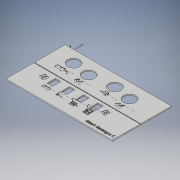
# Autodesk Inventor part: Caixa control - tapa
Saved by Autodesk Inventor 2019 (Build 230136000, 136)
## iProperties
Created: 2018-08-29
Part Number: Caixa control - tapa
Material: Genérico
Document SubType Name: Modeling
Designer: Albert Garangou Culebras
Density: 1 g/cm^3
Appearance: Valor por defecto
Author: Albert Garangou Culebras
Autodesk Inventor part; units mm, degrees
(part 1 of 2)
ref_plane "YZ Plane" through (0, 0, 0) normal (1, 0, 0) x (0, 1, 0)
ref_plane "XZ Plane" through (0, 0, 0) normal (0, 1, 0) x (-1, 0, 0)
ref_plane "XY Plane" through (0, 0, 0) normal (0, 0, 1) x (1, 0, 0)
sketch "Boceto1" plane through (0, 0, 0) normal (0, 1, 0) x (-1, 0, 0)
  line L0 (0, 0) -> (-180, 0)
  line L1 (-180, 0) -> (-180, -100)
  line L2 (-180, -100) -> (0, -100)
  line L3 (0, -100) -> (0, 0)
  dimension "d0" = 180
  dimension "d1" = 100
  constraints: 8 end point, 2 parallel, 1 horizontal, 1 perpendicular
  measures "d0" distance of L2.end L1.end
  measures "d1" distance of L1.end L0.end
extrude "base" add sketch "Boceto1" along normal blind 2
sketch "Boceto2" plane through (0, 2, 0) normal (0, 1, 0) x (1, 0, 0)
  line L0 (0, 100) -> (0, 0) projected
  line L1 (0, 0) -> (180, 0) projected
  line L2 (0, 100) -> (180, 100)
  line L3 (180, 100) -> (180, 0)
  line L4 (180, 0) -> (0, 0)
  line L5 (0, 0) -> (0, 100)
  line L6 (180, 50) -> (180, 0)
  line L7 (180, 0) -> (84.2308, 0)
  line L8 (180, 100) -> (0, 100) projected
  circle A0 centre (34.2888, 79.9235) radius 10.25
  circle A1 centre (104.2888, 79.9235) radius 10.25
  line L9 (50.4618, 35) -> (50.4618, 42)
  line L10 (50.4618, 42) -> (41.4618, 42)
  line L11 (41.4618, 42) -> (41.4618, 28)
  line L12 (41.4618, 28) -> (50.4618, 28)
  line L13 (50.4618, 28) -> (50.4618, 36)
  line L14 (65.4618, 35) -> (65.4618, 42)
  line L15 (65.4618, 42) -> (74.4618, 42)
  line L16 (74.4618, 42) -> (74.4618, 28)
  line L17 (74.4618, 28) -> (65.4618, 28)
  line L18 (65.4618, 28) -> (65.4618, 35)
  line L19 (89.4618, 35) -> (89.4618, 42)
  line L20 (89.4618, 42) -> (98.4618, 42)
  line L21 (98.4618, 42) -> (98.4618, 28)
  line L22 (98.4618, 28) -> (89.4618, 28)
  line L23 (89.4618, 28) -> (89.4618, 35)
  line L24 (113.4618, 42) -> (122.4618, 42)
  line L25 (122.4618, 42) -> (122.4618, 28)
  line L26 (122.4618, 28) -> (113.4618, 28)
  line L27 (113.4618, 28) -> (113.4618, 42)
  circle A2 centre (64.2888, 75.4263) radius 10.25
  circle A3 centre (134.2888, 74.9235) radius 10.25
  constraints: 50 end point, 11 perpendicular, 4 centre point, 4 parallel, 4 vertical, 3 horizontal, 3 point on line
sketch "Boceto3" plane through (0, 2, 0) normal (0, 1, 0) x (1, 0, 0)
  line L0 (35.7041, 64.3419) -> (35.7041, 63.6919)
  line L1 (35.7042, 59.1622) -> (35.7042, 59.8122)
  line L2 (37.6679, 61.7621) -> (37.6747, 62.4121)
  line L3 (37.6747, 62.4121) -> (38.9746, 62.3985)
  line L4 (37.6679, 61.7621) -> (37.6612, 61.1121)
  line L5 (37.6612, 61.1121) -> (38.961, 61.0986)
  line L6 (41.5539, 61.0919) -> (42.8539, 61.0919) construction
  line L7 (42.8539, 61.0919) -> (42.8539, 58.4716) construction
  spline S0 degree 2 poles (41.5539, 61.0919) (42.8539, 61.0919) (42.8539, 58.4716) knots 1 1 1 2 2 2
  line L8 (41.554, 62.3716) -> (44.1539, 62.3716) construction
  line L9 (44.1539, 62.3716) -> (44.1539, 58.4716) construction
  spline S1 degree 2 poles (41.554, 62.3716) (44.1539, 62.3716) (44.1539, 58.4716) knots 1 1 1 2 2 2
  line L10 (38.954, 61.0919) -> (41.554, 61.0919)
  line L11 (38.9541, 62.3919) -> (41.554, 62.3716)
  line L12 (37.6542, 60.4419) -> (35.7042, 60.4622)
  line L13 (37.6813, 63.0419) -> (35.7041, 63.0419)
  line L14 (37.6813, 63.0419) -> (37.6747, 62.4121)
  line L15 (37.6612, 61.1121) -> (37.6542, 60.4419)
  line L16 (42.8539, 57.8216) -> (44.1539, 57.8216)
  line L17 (44.1539, 57.8216) -> (44.1539, 58.4716)
  line L18 (44.1539, 57.8216) -> (43.8939, 57.8216)
  line L19 (42.8539, 58.4716) -> (42.8539, 57.8216)
  line L20 (58.9613, 57.27) -> (63.5735, 61.1094)
  line L21 (64.2117, 60.8104) -> (64.2117, 53.2631)
  line L22 (58.9754, 56.8292) -> (63.5531, 52.9999)
  arc A0 (63.5531, 52.9999) -> (64.2117, 53.2631) centre (63.7962, 53.3472) ccw
  arc A1 (64.2117, 60.8104) -> (63.5735, 61.1094) centre (63.7975, 60.7568) ccw
  arc A2 (58.9613, 57.27) -> (58.9754, 56.8292) centre (59.2258, 57.0578) ccw
  line L23 (64.4328, 57.3171) -> (69.0449, 61.1564)
  line L24 (69.6831, 60.8575) -> (69.6831, 53.3101)
  line L25 (64.4468, 56.8762) -> (69.0245, 53.0469)
  arc A3 (69.0245, 53.0469) -> (69.6831, 53.3101) centre (69.2676, 53.3943) ccw
  arc A4 (69.6831, 60.8575) -> (69.0449, 61.1564) centre (69.2689, 60.8039) ccw
  arc A5 (64.4328, 57.3171) -> (64.4468, 56.8762) centre (64.6972, 57.1049) ccw
  line L26 (58.9613, 57.27) -> (63.5735, 61.1094)
  line L27 (64.2117, 60.8104) -> (64.2117, 53.2631)
  line L28 (58.9754, 56.8292) -> (63.5531, 52.9999)
  arc A6 (58.9613, 57.27) -> (58.9754, 56.8292) centre (59.2258, 57.0578) ccw
  line L29 (69.6831, 60.8575) -> (69.6831, 53.3101)
  line L30 (64.4328, 57.3171) -> (69.0449, 61.1564)
  line L31 (64.4468, 56.8762) -> (69.0245, 53.0469)
  arc A7 (64.4328, 57.3171) -> (64.4468, 56.8762) centre (64.6972, 57.1049) ccw
  line L32 (128.7561, 56.7254) -> (133.3696, 60.5658)
  line L33 (134.0065, 60.2673) -> (134.0065, 52.7184)
  line L34 (128.7702, 56.2845) -> (133.3479, 52.4552)
  arc A8 (133.3479, 52.4552) -> (134.0065, 52.7184) centre (133.591, 52.8025) ccw
  arc A9 (128.7561, 56.7254) -> (128.7702, 56.2845) centre (129.0205, 56.5132) ccw
  line L35 (139.4779, 60.3128) -> (139.4779, 52.7655)
  arc A10 (138.8193, 52.5023) -> (139.4779, 52.7655) centre (139.0624, 52.8496) ccw
  line L36 (134.2275, 56.7724) -> (138.8397, 60.6118)
  line L37 (134.2416, 56.3316) -> (138.8193, 52.5023)
  arc A11 (134.2275, 56.7724) -> (134.2416, 56.3316) centre (134.4919, 56.5602) ccw
  arc A12 (134.0065, 60.2673) -> (133.3696, 60.5658) centre (133.618, 60.2673) ccw
  arc A13 (139.4779, 60.3128) -> (138.8397, 60.6118) centre (139.0799, 60.294) ccw
  arc A14 (101.959, 62.5573) -> (101.9701, 63.0852) centre (105.955, 62.7371) ccw
  spline S2 degree 3 poles (101.9701, 63.0852) (100.3792, 62.5267) (98.8482, 62.1984) (96.8436, 62.2447) knots 0 0 0 0 1 1 1 1
  circle A15 centre (105.955, 62.7371) radius 1
  arc A16 (108.9509, 62.892) -> (106.5532, 65.6768) centre (105.955, 62.7371) ccw
  line L38 (109.0736, 62.5385) -> (108.7201, 62.892)
  line L39 (109.0736, 62.5385) -> (109.4272, 62.892)
  arc A17 (109.2013, 62.892) -> (106.5532, 65.9315) centre (105.955, 62.7371) ccw
  line L40 (109.4272, 62.892) -> (109.2013, 62.892)
  line L41 (108.9509, 62.892) -> (108.7201, 62.892)
  line L42 (102.8865, 63.4069) -> (101.0538, 62.7635) construction
  arc A18 (101.2329, 62.8412) -> (102.6981, 63.3556) centre (94.8232, 83.4427) ccw construction
  line L43 (96.8436, 62.2447) -> (97.002, 61.7465)
  line L44 (106.5532, 65.9315) -> (106.5532, 65.6768)
  line L45 (35.7041, 64.3419) -> (35.7041, 64.4719)
  line L46 (35.7041, 64.3419) -> (35.7041, 65.6419)
  line L47 (35.7041, 65.6419) -> (33.7541, 65.6419)
  line L48 (33.7541, 65.6419) -> (33.7541, 64.3419)
  line L49 (33.7541, 64.3419) -> (22.7041, 64.3419)
  line L50 (22.7041, 59.1419) -> (22.7041, 64.3419)
  line L51 (33.7541, 59.1419) -> (33.7541, 57.8419)
  line L52 (33.7541, 57.8419) -> (35.704, 57.8419)
  line L53 (35.7042, 57.8419) -> (35.7042, 59.1622)
  line L54 (33.7541, 59.1419) -> (22.7041, 59.1419)
  line L55 (51.2122, 23.1412) -> (51.2122, 22.6162)
  line L56 (51.2122, 18.9576) -> (51.2122, 19.4826)
  line L57 (52.7873, 20.0076) -> (51.2122, 20.0076)
  line L58 (52.7872, 22.0912) -> (51.2122, 22.0912)
  line L59 (52.7872, 22.0912) -> (52.7872, 21.599)
  line L60 (52.7873, 20.549) -> (52.7873, 20.0076)
  line L61 (51.2122, 23.1412) -> (51.2122, 23.2462)
  line L62 (51.2122, 23.1412) -> (51.2122, 24.1912)
  line L63 (51.2122, 24.1912) -> (49.6372, 24.1912)
  line L64 (49.6372, 24.1912) -> (49.6372, 23.1412)
  line L65 (49.6372, 23.1412) -> (40.7122, 23.1412)
  line L66 (40.7122, 18.9412) -> (40.7122, 23.1412)
  line L67 (49.6372, 18.9412) -> (49.6372, 17.8912)
  line L68 (49.6372, 17.8912) -> (51.2122, 17.8912)
  line L69 (51.2122, 17.8912) -> (51.2122, 18.9576)
  line L70 (49.6372, 18.9412) -> (40.7122, 18.9412)
  line L71 (51.2122, 20.0076) -> (51.2122, 19.4826)
  line L72 (51.2122, 22.0912) -> (51.2122, 22.6162)
  line L73 (35.7042, 60.4622) -> (35.7042, 59.8122)
  line L74 (35.7041, 63.6919) -> (35.7041, 63.0419)
  line L75 (52.7872, 21.374) -> (52.4873, 21.374)
  line L76 (52.4873, 21.374) -> (52.4873, 20.774)
  line L77 (52.4873, 20.774) -> (52.7873, 20.774)
  line L78 (52.7873, 20.774) -> (52.7873, 20.549)
  line L79 (52.7872, 21.599) -> (52.7872, 21.374)
  line L80 (89.627, 23.9855) -> (97.277, 23.9855)
  line L81 (97.277, 16.3355) -> (89.627, 16.3355)
  line L82 (89.627, 16.3355) -> (89.627, 23.9855)
  line L83 (67.3452, 22.5763) -> (66.2952, 22.5763)
  line L84 (66.2952, 22.5763) -> (66.2952, 21.8763)
  line L85 (67.3452, 21.8763) -> (67.3452, 22.5763)
  line L86 (67.3452, 21.8763) -> (67.3452, 21.9463)
  line L87 (67.3452, 21.8763) -> (67.3452, 21.5263)
  line L88 (68.3953, 21.1763) -> (67.3452, 21.1763)
  line L89 (68.3953, 19.7747) -> (67.3452, 19.7763)
  line L90 (67.3452, 19.0763) -> (67.3452, 19.4263)
  line L91 (67.3452, 18.3653) -> (67.3452, 19.0763)
  line L92 (66.2952, 19.0749) -> (66.2952, 18.3749)
  line L93 (66.2952, 18.3749) -> (67.3452, 18.3749)
  line L94 (68.3953, 20.1357) -> (68.3953, 19.7747)
  line L95 (67.3452, 19.7763) -> (67.3452, 19.4263)
  line L96 (67.3452, 21.1763) -> (67.3452, 21.5263)
  line L97 (68.3953, 20.2857) -> (68.3953, 20.1357)
  line L98 (68.3953, 21.1763) -> (68.3953, 20.7878)
  line L99 (65.2366, 21.8749) -> (65.2366, 19.0749)
  line L100 (65.2366, 21.8763) -> (66.2952, 21.8763)
  line L101 (65.2366, 19.0749) -> (66.2952, 19.0749)
  line L102 (97.277, 23.9855) -> (97.277, 20.798)
  line L103 (97.277, 19.523) -> (97.277, 16.3355)
  line L104 (100.5679, 20.798) -> (100.5679, 19.523)
  line L105 (100.5679, 19.523) -> (97.277, 19.523)
  line L106 (97.277, 20.798) -> (100.5679, 20.798)
  line L107 (122.2298, 31.1299) -> (122.2298, 16.1299)
  line L108 (122.2298, 16.1299) -> (113.2298, 16.1299)
  line L109 (113.2298, 26.1299) -> (113.2298, 21.1299)
  line L110 (113.2298, 26.1299) -> (113.2298, 25.6299)
  line L111 (113.2298, 21.1299) -> (113.2298, 21.6299)
  line L112 (113.2298, 21.6299) -> (113.2298, 20.6299)
  line L113 (113.2298, 16.1299) -> (114.2298, 16.1299)
  line L114 (122.2298, 16.1299) -> (121.2298, 16.1299)
  line L115 (113.2298, 16.1299) -> (113.2298, 17.1299)
  line L116 (114.2298, 25.6299) -> (121.2298, 25.6299)
  line L117 (121.2298, 25.6299) -> (121.2298, 21.6299)
  line L118 (121.2298, 21.6299) -> (114.2298, 21.6299)
  line L119 (114.2298, 21.6299) -> (114.2298, 25.6299)
  line L120 (114.2298, 20.6299) -> (121.2298, 20.6299)
  line L121 (121.2298, 20.6299) -> (121.2298, 17.1299)
  line L122 (121.2298, 17.1299) -> (114.2298, 17.1299)
  line L123 (114.2298, 17.1299) -> (114.2298, 20.6299)
  line L124 (114.2298, 17.1299) -> (116.5298, 17.1299)
  line L125 (116.5298, 17.1299) -> (118.8298, 17.1299)
  line L126 (117.6798, 17.1299) -> (118.7948, 17.1299)
  line L127 (118.7948, 17.1299) -> (119.9098, 17.1299)
  line L128 (119.9098, 17.1299) -> (121.0248, 17.1299)
  circle A19 centre (120.4673, 19.4799) radius 0.45
  circle A20 centre (118.8673, 19.4799) radius 0.45
  circle A21 centre (117.2673, 19.4799) radius 0.45
  circle A22 centre (118.8673, 24.2799) radius 0.45
  circle A23 centre (120.4673, 24.2799) radius 0.45
  circle A24 centre (117.2673, 24.2799) radius 0.45
  circle A25 centre (118.8673, 29.0799) radius 0.45
  circle A26 centre (120.4673, 29.0799) radius 0.45
  circle A27 centre (117.2673, 29.0799) radius 0.45
  line L129 (114.2298, 17.1299) -> (114.2298, 18.1299)
  line L130 (114.2298, 17.1299) -> (114.9798, 17.1299)
  line L131 (114.9823, 17.6299) -> (117.0198, 17.6299)
  line L132 (117.0198, 17.6299) -> (117.0198, 18.1299)
  line L133 (117.0198, 18.1299) -> (114.9823, 18.1299)
  line L134 (114.9823, 18.1299) -> (114.9823, 17.6299)
  line L135 (114.9823, 22.6299) -> (114.9823, 22.1299)
  line L136 (114.9823, 22.1299) -> (117.0198, 22.1299)
  line L137 (117.0198, 22.6299) -> (114.9823, 22.6299)
  line L138 (117.0198, 22.1299) -> (117.0198, 22.6299)
  line L139 (114.9823, 27.6299) -> (114.9823, 27.1299)
  line L140 (117.0198, 27.6299) -> (114.9823, 27.6299)
  line L141 (117.0198, 27.1299) -> (117.0198, 27.6299)
  line L142 (114.9823, 27.1299) -> (117.0198, 27.1299)
  line L143 (121.2298, 30.6299) -> (121.2298, 26.6299)
  line L144 (40.7122, 23.1412) -> (40.7122, 18.9412)
  line L145 (49.6372, 18.9412) -> (40.7122, 18.9412)
  line L146 (49.6372, 18.9412) -> (49.6372, 17.8912)
  line L147 (49.6372, 17.8912) -> (51.2122, 17.8912)
  line L148 (51.2122, 17.8912) -> (51.2122, 20.0076)
  line L149 (51.2122, 20.0076) -> (52.7873, 20.0076)
  line L150 (52.7873, 20.0076) -> (52.7873, 20.774)
  line L151 (52.7873, 20.774) -> (52.4873, 20.774)
  line L152 (52.4873, 20.774) -> (52.4873, 21.3799)
  line L153 (52.4873, 21.3799) -> (52.7872, 21.3799)
  line L154 (52.7872, 21.3799) -> (52.7872, 22.0908)
  line L155 (52.7872, 22.0908) -> (51.2122, 22.0908)
  line L156 (51.2122, 22.0908) -> (51.2122, 24.1912)
  line L157 (49.6372, 24.1912) -> (51.2122, 24.1912)
  line L158 (49.6372, 24.1912) -> (49.6372, 23.1412)
  line L159 (49.6372, 23.1412) -> (40.7122, 23.1412)
  line L160 (40.7122, 23.1412) -> (40.7122, 18.9412)
  line L161 (22.7041, 64.3419) -> (22.7041, 59.1419)
  line L162 (22.7041, 59.1419) -> (33.7541, 59.1419)
  line L163 (33.7541, 57.8419) -> (33.7541, 59.1419)
  line L164 (33.7541, 57.8419) -> (35.7042, 57.8419)
  line L165 (35.7042, 57.8419) -> (35.7042, 60.4622)
  line L166 (35.7042, 60.4622) -> (37.6542, 60.4419)
  line L167 (37.6542, 60.4419) -> (37.6612, 61.1121)
  line L168 (37.6612, 61.1121) -> (37.6813, 63.0419)
  line L169 (37.6813, 63.0419) -> (35.7041, 63.0419)
  line L170 (35.7041, 63.0419) -> (35.7041, 65.6419)
  line L171 (35.7041, 65.6419) -> (33.7541, 65.6419)
  line L172 (33.7541, 65.6419) -> (33.7541, 64.3419)
  line L173 (33.7541, 64.3419) -> (22.7041, 64.3419)
  line L174 (22.7041, 64.3419) -> (22.7041, 59.1419)
  line L175 (42.8539, 57.8216) -> (44.1539, 57.8216)
  line L176 (44.1539, 58.4716) -> (44.1539, 57.8216)
  line L177 (42.8539, 58.4716) -> (42.8539, 57.8216)
  line L178 (41.554, 61.0919) -> (42.8539, 61.0919) construction
  line L179 (42.8539, 61.0919) -> (42.8539, 58.4716) construction
  spline S3 degree 2 poles (41.554, 61.0919) (42.8539, 61.0919) (42.8539, 58.4716) knots 1 1 1 2 2 2
  line L180 (41.554, 62.3716) -> (44.1539, 62.3716) construction
  line L181 (44.1539, 62.3716) -> (44.1539, 58.4716) construction
  spline S4 degree 2 poles (41.554, 62.3716) (44.1539, 62.3716) (44.1539, 58.4716) knots 1 1 1 2 2 2
  line L182 (65.2366, 21.8763) -> (65.2366, 19.0749)
  line L183 (66.2952, 19.0749) -> (65.2366, 19.0749)
  line L184 (66.2952, 19.0749) -> (66.2952, 18.3749)
  line L185 (66.2952, 18.3749) -> (67.3452, 18.3749)
  line L186 (67.3452, 18.3749) -> (67.3452, 19.7763)
  line L187 (67.3452, 19.7763) -> (68.3953, 19.7747)
  line L188 (68.3953, 20.2857) -> (68.3953, 19.7747)
  line L189 (68.3953, 20.7878) -> (68.3953, 21.1763)
  line L190 (68.3953, 21.1763) -> (67.3452, 21.1763)
  line L191 (67.3452, 21.1763) -> (67.3452, 22.5763)
  line L192 (67.3452, 22.5763) -> (66.2952, 22.5763)
  line L193 (66.2952, 22.5763) -> (66.2952, 21.8763)
  line L194 (66.2952, 21.8763) -> (65.2366, 21.8763)
  line L195 (65.2366, 21.8763) -> (65.2366, 19.0749)
  spline S5 degree 3 poles (68.3953, 20.7878) (70.7304, 20.7878) (70.1192, 19.8403) (75.3334, 20.4894) knots 0 0 0 0 1 1 1 1
  line L196 (75.3828, 20.0925) -> (75.3334, 20.4894)
  line L197 (91.5068, 17.6299) -> (92.143, 17.6299)
  line L198 (92.143, 17.6299) -> (92.143, 22.0105)
  line L199 (92.143, 22.0105) -> (93.452, 19.0299)
  line L200 (93.452, 19.0299) -> (93.8546, 19.0299)
  line L201 (93.8546, 19.0299) -> (95.1799, 22.0105)
  line L202 (95.1799, 22.0105) -> (95.1799, 17.6299)
  line L203 (95.1799, 17.6299) -> (95.8762, 17.6299)
  line L204 (95.8762, 17.6299) -> (95.8762, 22.7264)
  line L205 (94.9375, 22.7264) -> (93.6941, 19.9299)
  line L206 (93.6941, 19.9299) -> (92.4659, 22.7264)
  line L207 (91.5068, 22.7264) -> (92.4659, 22.7264)
  line L208 (91.5068, 22.7264) -> (91.5068, 17.6299)
  line L209 (94.9375, 22.7264) -> (95.8762, 22.7264)
  line L210 (113.2298, 20.6299) -> (113.2298, 17.1299)
  line L211 (114.2298, 26.6299) -> (113.2298, 26.6299)
  line L212 (113.2298, 26.6299) -> (113.2298, 26.1299)
  line L213 (114.2298, 26.6299) -> (122.2298, 26.6299)
  line L214 (37.6612, 61.1121) -> (37.6747, 62.4121)
  line L215 (68.3953, 20.7878) -> (68.3953, 20.3878)
  line L216 (68.3953, 20.3878) -> (68.3953, 19.7747)
  spline S6 degree 5 poles (101.959, 62.5573) (101.0032, 62.2312) (100.028, 61.9616) (99.0225, 61.7956) (98.0118, 61.7336) (97.002, 61.7465) knots 0 0 0 0 0 0 1 1 1 1 1 1
  spline S7 degree 5 poles (68.3953, 20.3878) (68.7147, 20.3874) (69.0333, 20.3731) (69.3537, 20.3357) (70.0075, 20.1748) (70.6566, 19.9957) (71.0075, 19.9367) (72.0927, 19.8215) (73.1869, 19.8682) (73.9195, 19.924) (74.6525, 20.0016) (75.3828, 20.0925) knots 0 0 0 0 0 0 0.226556 0.226556 0.226556 0.477707 0.477707 0.477707 1 1 1 1 1 1
  point P0 (0, 0)
  point P1 (126.2308, 70)
  point P2 (69.8531, 20.6216)
  point P3 (70.8387, 20.3848)
  point P4 (117.6798, 19.4799)
  point P5 (117.6798, 24.2799)
  point P6 (117.6798, 29.0799)
  dimension "d288" = 0.4
  dimension "d259" = 1.6
  dimension "d266" = 4.8
  dimension "d276" = 4.5
  dimension "d283" = 5
  dimension "d289" = 1
  constraints: 418 end point, 42 vertical, 36 collinear, 35 point on circle, 34 perpendicular, 28 centre point, 20 point on line, 12 horizontal, 11 parallel, 5 coincident, 3 midpoint, 1 tangent, 64 other
  measures "d259" distance of A19.centre A20.centre
  measures "d266" distance of A21.centre A24.centre
  measures "d276" distance of L131.start L135.end
  measures "d283" distance of L135.start L139.start
  measures "d289" distance of L116.start L211.start
extrude "Extrusión3" cut sketch "Boceto3" against normal blind 0.5 contours L0 L74 L13 L14 L2 L4 L15 L12 L73 L1 L53 L52 L51 L54 L50 L49 L48 L47 L46 L45 | L20 A1 L21 A0 L22 A2 | L23 A4 L24 A3 L25 A5 | L32 A12 L33 A8 L34 A9 | L35 A10 L37 A11 L36 A13 | S6 L43 S2 A14 | L55 L72 L58 L59 L79 L153 L152 L76 L77 L78 L60 L57 L71 L56 L69 L68 L67 L70 L66 L65 L64 L63 L62 L61 | L80 L102 L106 L104 L105 L103 L81 L82 | L85 L87 L96 L88 L98 L215 L216 L97 L94 L89 L95 L90 L91 L93 L92 L101 L99 L100 L84 L83 | S5 L196 S7 L215 | L107 L108 L115 L210 L112 L109 L212 L211 L213 | A19 | A20 | A21 | A22 | A23 | A24 | L134 L133 L132 L131 | L137 L138 L136 L135
sketch "Boceto5" plane through (0, 2, 0) normal (0, 1, 0) x (1, 0, 0)
  line L0 (37.6813, 63.0419) -> (37.6542, 60.4419) projected
  line L1 (37.6747, 62.4093) -> (37.6612, 61.1175)
  line L2 (41.6533, 62.4093) -> (37.6747, 62.4093)
  line L3 (41.6533, 62.4093) -> (44.1386, 62.4093) construction
  line L4 (44.1386, 62.4093) -> (44.1386, 58.5428) construction
  spline S0 degree 2 poles (41.6533, 62.4093) (44.1386, 62.4093) (44.1386, 58.5428) knots 1 1 1 2 2 2
  line L5 (41.6533, 61.1175) -> (42.896, 61.1175) construction
  line L6 (42.896, 61.1175) -> (42.896, 58.5428) construction
  spline S1 degree 2 poles (41.6533, 61.1175) (42.896, 61.1175) (42.896, 58.5428) knots 1 1 1 2 2 2
  line L7 (42.896, 58.5428) -> (44.1386, 58.5428)
  line L8 (37.6612, 61.1175) -> (41.6533, 61.1175)
  point P0 (0, 0)
  constraints: 8 end point, 3 horizontal, 2 point on line, 2 vertical, 6 other
extrude "Extrusión4" cut sketch "Boceto5" against normal blind 0.5
sketch "Boceto6" plane through (0, 2, 0) normal (0, 1, 0) x (1, 0, 0)
  spline S0 degree 4 poles (29.0799, 35.9708) (29.157, 35.7147) (29.5973, 35.6307) (29.6514, 35.9754) (29.6224, 36.5115) (30.003, 37.3994) (30.9963, 38.6611) (31.8038, 39.1799) (34.1243, 38.5401) (34.4092, 36.16) knots 0 0 0 0 0 0.168165 0.246229 0.343173 0.454491 0.580711 1 1 1 1 1
  spline S1 degree 4 poles (34.4092, 36.16) (34.7426, 35.3106) (32.7275, 33.2427) (32.5523, 36.2152) (30.5175, 34.9657) knots 0 0 0 0 0 1 1 1 1 1
  spline S2 degree 3 poles (30.5175, 34.9657) (30.1475, 33.8706) (31.9148, 35.589) (33.3235, 32.8129) knots 0 0 0 0 1 1 1 1
  spline S3 degree 4 poles (29.2384, 33.5854) (28.9713, 32.822) (29.1745, 27.8691) (22.2619, 31.4963) (24.9254, 34.4527) knots 0 0 0 0 0 1 1 1 1 1
  spline S4 degree 3 poles (24.9254, 34.4527) (25.3025, 34.7607) (26.1651, 34.7965) (26.8468, 34.2785) knots 0 0 0 0 1 1 1 1
  spline S5 degree 3 poles (28.1827, 34.9339) (27.2948, 35.0506) (26.5081, 35.3521) (25.9075, 36.0652) knots 0 0 0 0 1 1 1 1
  spline S6 degree 3 poles (29.2384, 38.9749) (29.7153, 38.8274) (29.0086, 37.0279) (28.8371, 37.2609) knots 0 0 0 0 1 1 1 1
  spline S7 degree 2 poles (28.9441, 37.2803) (28.8501, 36.3273) (29.0799, 35.9708) knots 0 0 0 1 1 1
  spline S8 degree 4 poles (25.9075, 36.0652) (25.5031, 36.2597) (25.0892, 37.4783) (25.8437, 39.2045) (28.412, 40.2658) (29.5743, 39.0581) (29.3681, 38.316) knots 0 0 0 0 0 0.38825 0.566915 1 1 1 1 1
  spline S9 degree 2 poles (28.1827, 34.9339) (28.2241, 34.93) (28.2695, 34.9084) knots 0 0 0 1 1 1
  line L0 (28.247, 34.9191) -> (28.2921, 34.8978) construction
  arc A0 (28.2873, 34.8994) -> (28.2513, 34.9165) centre (28.117, 34.5869) ccw construction
  spline S10 degree 4 poles (26.8468, 34.2785) (26.8742, 34.2176) (27.9219, 34.0143) (28.7341, 34.5531) (28.2695, 34.9084) knots 0 0 0 0 0 1 1 1 1 1
  line L1 (29.5064, 33.6433) -> (30.5358, 34.5853)
  line L2 (30.5358, 34.5853) -> (29.4747, 35.7449)
  line L3 (28.2695, 34.4831) -> (29.4747, 35.7449)
  line L4 (28.349, 34.5722) -> (29.2384, 33.5854)
  spline S11 degree 3 poles (29.2384, 33.5854) (29.464, 33.9116) (30.057, 33.5762) (30.0053, 32.599) knots 0 0 0 0 1 1 1 1
  spline S12 degree 4 poles (30.0053, 32.599) (29.9904, 32.3205) (29.8007, 31.7908) (29.1962, 30.9163) (29.973, 30.0496) (30.9102, 29.5496) (31.4961, 29.9491) (33.4717, 30.4348) (33.5063, 32.1817) knots 0 0 0 0 0 0.268483 0.383338 0.491913 0.605909 1 1 1 1 1
  spline S13 degree 2 poles (33.5063, 32.1817) (33.5448, 32.5565) (33.3235, 32.8129) knots 0 0 0 1 1 1
  point P0 (0, 0)
  point P1 (29.3679, 35.7325)
  point P2 (29.5571, 35.8001)
  point P3 (29.6292, 36.0072)
  point P4 (29.6563, 36.381)
  point P5 (29.9672, 37.2278)
  point P6 (30.607, 38.1197)
  point P7 (31.2874, 38.6375)
  point P8 (32.4634, 38.7049)
  point P9 (34.1759, 35.2829)
  point P10 (33.3695, 34.7967)
  point P11 (32.3652, 35.0292)
  point P12 (31.0767, 34.531)
  point P13 (28.9716, 32.4514)
  point P14 (27.7552, 30.9492)
  point P15 (25.3435, 31.3256)
  point P16 (25.3271, 34.6378)
  point P17 (25.9996, 34.6497)
  point P18 (27.3265, 35.1223)
  point P19 (26.5793, 35.473)
  point P20 (28.9491, 36.3444)
  point P21 (25.4859, 36.6468)
  point P22 (25.4514, 37.779)
  point P23 (26.174, 38.9117)
  point P24 (27.6829, 39.6636)
  point P25 (29.0092, 39.3066)
  point P26 (26.9393, 34.2428)
  point P27 (27.6806, 34.2429)
  point P28 (29.4493, 33.7062)
  point P29 (29.7406, 33.5661)
  point P30 (29.9059, 32.1623)
  point P31 (29.6292, 31.4538)
  point P32 (29.5571, 30.7017)
  point P33 (30.0211, 30.0807)
  point P34 (30.5358, 29.8089)
  point P35 (31.0074, 29.7895)
  point P36 (32.0167, 30.1098)
  point P37 (33.4771, 32.536)
  constraints: 10 end point, 2 midpoint, 1 centre point, 1 perpendicular, 1 point on circle, 73 other
sketch "Boceto8" plane through (0, 2, 0) normal (0, 1, 0) x (1, 0, 0)
  spline S0 degree 4 poles (133.7635, 35.9708) (133.8407, 35.7147) (134.281, 35.6307) (134.3351, 35.9754) (134.306, 36.5115) (134.6867, 37.3994) (135.6799, 38.6611) (136.4874, 39.1799) (138.808, 38.5401) (139.0929, 36.16) knots 0 0 0 0 0 0.168165 0.246229 0.343173 0.454491 0.580711 1 1 1 1 1
  spline S1 degree 4 poles (139.0929, 36.16) (139.4262, 35.3106) (137.4111, 33.2428) (137.2359, 36.2152) (135.2011, 34.9657) knots 0 0 0 0 0 1 1 1 1 1
  spline S2 degree 3 poles (135.2011, 34.9657) (134.8312, 33.8706) (136.5984, 35.589) (138.0072, 32.8129) knots 0 0 0 0 1 1 1 1
  spline S3 degree 4 poles (134.6889, 32.599) (134.6741, 32.3205) (134.4844, 31.7908) (133.8799, 30.9164) (134.6567, 30.0496) (135.5938, 29.5497) (136.1798, 29.9491) (138.1553, 30.4347) (138.19, 32.1817) knots 0 0 0 0 0 0.268481 0.383336 0.491911 0.605908 1 1 1 1 1
  spline S4 degree 2 poles (138.19, 32.1817) (138.2281, 32.5568) (138.0072, 32.8129) knots 0 0 0 1 1 1
  spline S5 degree 3 poles (133.9221, 33.5854) (134.1353, 33.9306) (134.7352, 33.5812) (134.6889, 32.599) knots 0 0 0 0 1 1 1 1
  line L0 (134.19, 33.6433) -> (135.2195, 34.5853)
  line L1 (135.2195, 34.5853) -> (134.1584, 35.7449)
  spline S6 degree 2 poles (132.8663, 34.9339) (132.9078, 34.93) (132.9532, 34.9084) knots 0 0 0 1 1 1
  line L2 (132.9307, 34.9191) -> (132.9757, 34.8978) construction
  arc A0 (132.971, 34.8994) -> (132.935, 34.9165) centre (132.8007, 34.5869) ccw construction
  line L3 (132.9532, 34.4831) -> (134.1584, 35.7449)
  spline S7 degree 4 poles (133.9221, 33.5854) (133.6546, 32.8232) (133.8613, 27.8633) (126.9409, 31.5047) (129.6091, 34.4527) knots 0 0 0 0 0 1 1 1 1 1
  spline S8 degree 4 poles (131.5305, 34.2785) (131.5578, 34.2176) (132.6056, 34.0143) (133.4177, 34.5531) (132.9532, 34.9084) knots 0 0 0 0 0 1 1 1 1 1
  line L4 (133.0326, 34.5722) -> (133.9221, 33.5854)
  spline S9 degree 3 poles (129.6091, 34.4527) (129.9861, 34.7608) (130.8488, 34.7962) (131.5305, 34.2785) knots 0 0 0 0 1 1 1 1
  spline S10 degree 3 poles (132.8663, 34.9339) (131.9785, 35.0507) (131.1917, 35.3522) (130.5912, 36.0652) knots 0 0 0 0 1 1 1 1
  spline S11 degree 3 poles (133.9221, 38.9749) (134.3989, 38.8274) (133.6923, 37.0279) (133.5207, 37.2609) knots 0 0 0 0 1 1 1 1
  spline S12 degree 2 poles (133.6277, 37.2803) (133.5398, 36.3224) (133.7635, 35.9708) knots 0 0 0 1 1 1
  spline S13 degree 4 poles (130.5912, 36.0652) (130.1868, 36.2595) (129.7733, 37.4779) (130.5282, 39.2035) (133.0957, 40.2649) (134.2582, 39.0581) (134.0518, 38.316) knots 0 0 0 0 0 0.388238 0.566914 1 1 1 1 1
  spline S14 degree 4 poles (29.0799, 35.9708) (29.157, 35.7147) (29.5973, 35.6307) (29.6514, 35.9754) (29.6224, 36.5115) (30.003, 37.3994) (30.9963, 38.6611) (31.8038, 39.1799) (34.1243, 38.5401) (34.4092, 36.16) knots 0 0 0 0 0 0.168165 0.246229 0.343173 0.454491 0.580711 1 1 1 1 1
  spline S15 degree 4 poles (34.4092, 36.16) (34.7426, 35.3106) (32.7275, 33.2427) (32.5523, 36.2152) (30.5175, 34.9657) knots 0 0 0 0 0 1 1 1 1 1
  spline S16 degree 3 poles (30.5175, 34.9657) (30.1475, 33.8706) (31.9148, 35.589) (33.3235, 32.8129) knots 0 0 0 0 1 1 1 1
  spline S17 degree 4 poles (29.2384, 33.5854) (28.9712, 32.8222) (29.1751, 27.8679) (22.2609, 31.4979) (24.9254, 34.4527) knots 0 0 0 0 0 1 1 1 1 1
  spline S18 degree 3 poles (24.9254, 34.4527) (25.3025, 34.7607) (26.1651, 34.7965) (26.8468, 34.2785) knots 0 0 0 0 1 1 1 1
  spline S19 degree 3 poles (28.1827, 34.9339) (27.2948, 35.0506) (26.5081, 35.3522) (25.9075, 36.0652) knots 0 0 0 0 1 1 1 1
  spline S20 degree 3 poles (29.2384, 38.9749) (29.7153, 38.8274) (29.0086, 37.0279) (28.8371, 37.2609) knots 0 0 0 0 1 1 1 1
  spline S21 degree 2 poles (28.9441, 37.2803) (28.8512, 36.3264) (29.0799, 35.9708) knots 0 0 0 1 1 1
  spline S22 degree 4 poles (25.9075, 36.0652) (25.5031, 36.2597) (25.0893, 37.4782) (25.8438, 39.2043) (28.412, 40.2656) (29.5744, 39.0581) (29.3681, 38.316) knots 0 0 0 0 0 0.388248 0.566915 1 1 1 1 1
  spline S23 degree 2 poles (28.1827, 34.9339) (28.2241, 34.93) (28.2695, 34.9084) knots 0 0 0 1 1 1
  line L5 (28.247, 34.9191) -> (28.2921, 34.8978) construction
  arc A1 (28.2873, 34.8994) -> (28.2513, 34.9165) centre (28.117, 34.5869) ccw construction
  spline S24 degree 4 poles (26.8468, 34.2785) (26.8742, 34.2176) (27.9219, 34.0143) (28.7341, 34.5531) (28.2695, 34.9084) knots 0 0 0 0 0 1 1 1 1 1
  line L6 (29.5064, 33.6433) -> (30.5358, 34.5853)
  line L7 (30.5358, 34.5853) -> (29.4747, 35.7449)
  line L8 (28.2695, 34.4831) -> (29.4747, 35.7449)
  line L9 (28.349, 34.5722) -> (29.2384, 33.5854)
  spline S25 degree 3 poles (29.2384, 33.5854) (29.4617, 33.9151) (30.0559, 33.5771) (30.0053, 32.599) knots 0 0 0 0 1 1 1 1
  spline S26 degree 4 poles (30.0053, 32.599) (29.9904, 32.3205) (29.8007, 31.7908) (29.1962, 30.9163) (29.973, 30.0496) (30.9102, 29.5496) (31.4961, 29.9491) (33.4717, 30.4348) (33.5063, 32.1817) knots 0 0 0 0 0 0.268483 0.383338 0.491912 0.605909 1 1 1 1 1
  spline S27 degree 2 poles (33.5063, 32.1817) (33.5447, 32.5565) (33.3235, 32.8129) knots 0 0 0 1 1 1
  point P0 (0, 0)
  point P1 (134.0516, 35.7325)
  point P2 (134.2407, 35.8001)
  point P3 (134.3129, 36.0072)
  point P4 (134.34, 36.381)
  point P5 (134.6509, 37.2278)
  point P6 (135.2907, 38.1197)
  point P7 (135.9711, 38.6375)
  point P8 (137.147, 38.7049)
  point P9 (138.8595, 35.2829)
  point P10 (138.0532, 34.7967)
  point P11 (137.0489, 35.0292)
  point P12 (135.7604, 34.531)
  point P13 (134.5896, 32.1623)
  point P14 (134.3129, 31.4539)
  point P15 (134.2407, 30.7018)
  point P16 (134.7047, 30.0807)
  point P17 (135.2195, 29.809)
  point P18 (135.691, 29.7896)
  point P19 (136.7003, 30.1098)
  point P20 (138.1606, 32.5363)
  point P21 (133.6554, 32.4512)
  point P22 (134.4148, 33.578)
  point P23 (134.1261, 33.7147)
  point P24 (132.439, 30.949)
  point P25 (132.3643, 34.2429)
  point P26 (130.0246, 31.3286)
  point P27 (131.623, 34.2428)
  point P28 (132.0102, 35.1223)
  point P29 (130.0107, 34.6379)
  point P30 (130.6833, 34.6497)
  point P31 (131.2629, 35.4731)
  point P32 (133.6361, 36.3391)
  point P33 (130.1698, 36.6465)
  point P34 (133.6931, 39.3062)
  point P35 (130.1355, 37.7783)
  point P36 (132.3671, 39.6629)
  point P37 (130.8582, 38.9109)
  point P38 (29.3679, 35.7325)
  point P39 (29.5571, 35.8001)
  point P40 (29.6292, 36.0072)
  point P41 (29.6563, 36.381)
  point P42 (29.9672, 37.2278)
  point P43 (30.607, 38.1197)
  point P44 (31.2874, 38.6375)
  point P45 (32.4634, 38.7049)
  point P46 (34.1759, 35.2829)
  point P47 (33.3695, 34.7967)
  point P48 (32.3652, 35.0292)
  point P49 (31.0767, 34.531)
  point P50 (28.9716, 32.4514)
  point P51 (27.7552, 30.9491)
  point P52 (25.343, 31.3262)
  point P53 (25.3271, 34.6378)
  point P54 (25.9996, 34.6497)
  point P55 (27.3265, 35.1223)
  point P56 (26.5793, 35.473)
  point P57 (28.9497, 36.3434)
  point P58 (25.4859, 36.6468)
  point P59 (25.4515, 37.7789)
  point P60 (26.1741, 38.9116)
  point P61 (27.683, 39.6635)
  point P62 (29.0092, 39.3066)
  point P63 (26.9393, 34.2428)
  point P64 (27.6806, 34.2429)
  point P65 (29.448, 33.7077)
  point P66 (29.7388, 33.5683)
  point P67 (29.9059, 32.1623)
  point P68 (29.6292, 31.4538)
  point P69 (29.557, 30.7018)
  point P70 (30.0211, 30.0807)
  point P71 (30.5358, 29.8089)
  point P72 (31.0074, 29.7895)
  point P73 (32.0167, 30.1098)
  point P74 (33.4771, 32.536)
  constraints: 20 end point, 4 midpoint, 2 centre point, 2 perpendicular, 2 point on circle, 146 other
extrude "Extrusión6" cut sketch "Boceto8" against normal blind 0.5 contours S0 L3 L4 S8 S6 S10 S13 S11 S12 | S0 S1 S2 L1 | L1 S2 L0 S5 L4 L3 | L4 S7 S9 S8 L3 | S11 S13 | S2 S4 S3 S5 L0 picked at (134.0684, 38.4188)
extrude "Extrusión7" cut sketch "Boceto6" against normal blind 0.5 contours S0 L3 L4 S10 S9 S5 S8 S6 S7 | S0 S1 S2 L2 | L2 S2 L1 S11 L4 L3 | L2 S2 | L4 S3 S4 S10 L3 | S2 S13 S12 S11 L1
sketch "Boceto10" plane through (0, 2, 0) normal (0, 1, 0) x (1, 0, 0)
  line L0 (128.9902, 8.9769) -> (181.2554, 8.9769) construction
  line L1 (181.2554, 8.9769) -> (181.2554, -0.3757) construction
  line L2 (181.2554, -0.3757) -> (128.9902, -0.3757) construction
  line L3 (128.9902, -0.3757) -> (128.9902, 8.9769) construction
  line L4 (128.9624, 4.4852) -> (130.4119, 8.7852)
  line L5 (130.4119, 8.7852) -> (131.1158, 8.7852)
  line L6 (131.1158, 8.7852) -> (132.5654, 4.4852)
  line L7 (132.5654, 4.4852) -> (131.9626, 4.4852)
  line L8 (131.9626, 4.4852) -> (131.5723, 5.6874)
  line L9 (131.5723, 5.6874) -> (129.9311, 5.6874)
  line L10 (129.9311, 5.6874) -> (129.5408, 4.4852)
  line L11 (129.5408, 4.4852) -> (128.9624, 4.4852)
  line L12 (131.4155, 6.1752) -> (130.75, 8.1998)
  line L13 (130.75, 8.1998) -> (130.0879, 6.1752)
  line L14 (130.0879, 6.1752) -> (131.4155, 6.1752)
  line L15 (133.4854, 4.4852) -> (132.9418, 4.4852)
  line L16 (132.9418, 4.4852) -> (132.9418, 8.9769)
  line L17 (132.9418, 8.9769) -> (133.4854, 8.9769)
  line L18 (133.4854, 8.9769) -> (133.4854, 4.4852)
  spline S0 degree 2 poles (136.9874, 6.1508) (136.9874, 5.3598) (136.2208, 4.3946) (135.6423, 4.3946) knots 0 0 0 1 2 2 2
  spline S1 degree 2 poles (135.6423, 4.3946) (135.381, 4.3946) (135.0081, 4.5235) (134.8269, 4.635) knots 0 0 0 1 2 2 2
  line L19 (134.8269, 4.635) -> (134.7921, 4.4852)
  line L20 (134.7921, 4.4852) -> (134.2833, 4.4852)
  line L21 (134.2833, 4.4852) -> (134.2833, 8.9769)
  line L22 (134.2833, 8.9769) -> (134.8269, 8.9769)
  line L23 (134.8269, 8.9769) -> (134.8269, 7.3739)
  spline S2 degree 2 poles (134.8269, 7.3739) (135.0325, 7.5586) (135.5099, 7.8025) (135.8131, 7.8025) knots 0 0 0 1 2 2 2
  spline S3 degree 2 poles (135.8131, 7.8025) (136.3602, 7.8025) (136.9874, 6.9279) (136.9874, 6.1508) knots 0 0 0 1 2 2 2
  spline S4 degree 2 poles (136.4264, 6.109) (136.4264, 6.6875) (136.0744, 7.2868) (135.6842, 7.2868) knots 0 0 0 1 2 2 2
  spline S5 degree 2 poles (135.6842, 7.2868) (135.4646, 7.2868) (135.0116, 7.0777) (134.8269, 6.9175) knots 0 0 0 1 2 2 2
  line L24 (134.8269, 6.9175) -> (134.8269, 5.0671)
  spline S6 degree 2 poles (134.8269, 5.0671) (135.0325, 4.9661) (135.3496, 4.8824) (135.5378, 4.8824) knots 0 0 0 1 2 2 2
  spline S7 degree 2 poles (135.5378, 4.8824) (135.9525, 4.8824) (136.4264, 5.4713) (136.4264, 6.109) knots 0 0 0 1 2 2 2
  spline S8 degree 2 poles (138.9527, 4.412) (138.1791, 4.412) (137.3289, 5.2797) (137.3289, 6.0812) knots 0 0 0 1 2 2 2
  spline S9 degree 2 poles (137.3289, 6.0812) (137.3289, 6.8687) (138.1547, 7.8025) (138.8203, 7.8025) knots 0 0 0 1 2 2 2
  spline S10 degree 2 poles (138.8203, 7.8025) (139.12, 7.8025) (139.5834, 7.6283) (139.7542, 7.4436) knots 0 0 0 1 2 2 2
  spline S11 degree 2 poles (139.7542, 7.4436) (139.9284, 7.2589) (140.1131, 6.7258) (140.1131, 6.339) knots 0 0 0 1 2 2 2
  line L25 (140.1131, 6.339) -> (140.1131, 6.0428)
  line L26 (140.1131, 6.0428) -> (137.8795, 6.0428)
  spline S12 degree 2 poles (137.8795, 6.0428) (137.8795, 5.4818) (138.444, 4.8859) (138.9457, 4.8859) knots 0 0 0 1 2 2 2
  spline S13 degree 2 poles (138.9457, 4.8859) (139.1235, 4.8859) (139.4684, 4.9661) (139.6078, 5.0288) knots 0 0 0 1 2 2 2
  spline S14 degree 2 poles (139.6078, 5.0288) (139.7542, 5.0985) (139.9563, 5.2205) (140.0225, 5.2762) knots 0 0 0 1 2 2 2
  line L27 (140.0225, 5.2762) -> (140.0538, 5.2762)
  line L28 (140.0538, 5.2762) -> (140.0538, 4.6838)
  spline S15 degree 2 poles (140.0538, 4.6838) (139.9598, 4.6455) (139.674, 4.534) (139.5625, 4.5026) knots 0 0 0 1 2 2 2
  spline S16 degree 2 poles (139.5625, 4.5026) (139.4057, 4.4573) (139.1478, 4.412) (138.9527, 4.412) knots 0 0 0 1 2 2 2
  spline S17 degree 2 poles (139.5834, 6.4575) (139.5765, 6.677) (139.4859, 6.9976) (139.3987, 7.1056) knots 0 0 0 1 2 2 2
  spline S18 degree 2 poles (139.3987, 7.1056) (139.3047, 7.2276) (139.0085, 7.3565) (138.7889, 7.3565) knots 0 0 0 1 2 2 2
  spline S19 degree 2 poles (138.7889, 7.3565) (138.5729, 7.3565) (138.2697, 7.2276) (138.1443, 7.1021) knots 0 0 0 1 2 2 2
  spline S20 degree 2 poles (138.1443, 7.1021) (138.0223, 6.9732) (137.8969, 6.6631) (137.8795, 6.4575) knots 0 0 0 1 2 2 2
  line L29 (137.8795, 6.4575) -> (139.5834, 6.4575)
  line L30 (142.3746, 7.13) -> (142.3467, 7.13)
  spline S21 degree 2 poles (142.3467, 7.13) (142.284, 7.1474) (142.1481, 7.1544) (142.054, 7.1544) knots 0 0 0 1 2 2 2
  spline S22 degree 2 poles (142.054, 7.1544) (141.8345, 7.1544) (141.4024, 6.9628) (141.2072, 6.7746) knots 0 0 0 1 2 2 2
  line L31 (141.2072, 6.7746) -> (141.2072, 4.4852)
  line L32 (141.2072, 4.4852) -> (140.6637, 4.4852)
  line L33 (140.6637, 4.4852) -> (140.6637, 7.7119)
  line L34 (140.6637, 7.7119) -> (141.2072, 7.7119)
  line L35 (141.2072, 7.7119) -> (141.2072, 7.2311)
  spline S23 degree 2 poles (141.2072, 7.2311) (141.5034, 7.4959) (141.946, 7.7119) (142.1551, 7.7119) knots 0 0 0 1 2 2 2
  spline S24 degree 2 poles (142.1551, 7.7119) (142.2387, 7.7119) (142.3223, 7.705) (142.3746, 7.6945) knots 0 0 0 1 2 2 2
  line L36 (142.3746, 7.6945) -> (142.3746, 7.13)
  spline S25 degree 2 poles (143.7719, 4.4225) (143.3294, 4.4225) (142.8311, 4.9277) (142.8311, 5.4748) knots 0 0 0 1 2 2 2
  line L37 (142.8311, 5.4748) -> (142.8311, 7.2624)
  line L38 (142.8311, 7.2624) -> (142.4652, 7.2624)
  line L39 (142.4652, 7.2624) -> (142.4652, 7.7119)
  line L40 (142.4652, 7.7119) -> (142.8311, 7.7119)
  line L41 (142.8311, 7.7119) -> (142.8311, 8.6389)
  line L42 (142.8311, 8.6389) -> (143.3747, 8.6389)
  line L43 (143.3747, 8.6389) -> (143.3747, 7.7119)
  line L44 (143.3747, 7.7119) -> (144.3748, 7.7119)
  line L45 (144.3748, 7.7119) -> (144.3748, 7.2624)
  line L46 (144.3748, 7.2624) -> (143.3747, 7.2624)
  line L47 (143.3747, 7.2624) -> (143.3747, 5.7257)
  spline S26 degree 2 poles (143.3747, 5.7257) (143.3747, 5.4818) (143.3921, 5.2135) (143.4513, 5.0985) knots 0 0 0 1 2 2 2
  spline S27 degree 2 poles (143.4513, 5.0985) (143.5001, 4.9974) (143.7196, 4.8964) (143.9078, 4.8964) knots 0 0 0 1 2 2 2
  spline S28 degree 2 poles (143.9078, 4.8964) (144.0402, 4.8964) (144.2876, 4.9765) (144.3434, 5.0009) knots 0 0 0 1 2 2 2
  line L48 (144.3434, 5.0009) -> (144.3748, 5.0009)
  line L49 (144.3748, 5.0009) -> (144.3748, 4.5131)
  spline S29 degree 2 poles (144.3748, 4.5131) (144.2214, 4.4713) (143.9078, 4.4225) (143.7719, 4.4225) knots 0 0 0 1 2 2 2
  spline S30 degree 2 poles (148.4657, 4.4016) (148.0092, 4.4016) (147.253, 4.6803) (146.9812, 4.9626) knots 0 0 0 1 2 2 2
  spline S31 degree 2 poles (146.9812, 4.9626) (146.7094, 5.2483) (146.4202, 6.0916) (146.4202, 6.6387) knots 0 0 0 1 2 2 2
  spline S32 degree 2 poles (146.4202, 6.6387) (146.4202, 7.1579) (146.7129, 7.9803) (146.9847, 8.273) knots 0 0 0 1 2 2 2
  spline S33 degree 2 poles (146.9847, 8.273) (147.2461, 8.5552) (148.0127, 8.8619) (148.4692, 8.8619) knots 0 0 0 1 2 2 2
  spline S34 degree 2 poles (148.4692, 8.8619) (148.6887, 8.8619) (149.0859, 8.7991) (149.2671, 8.7434) knots 0 0 0 1 2 2 2
  spline S35 degree 2 poles (149.2671, 8.7434) (149.4135, 8.7016) (149.7689, 8.5483) (149.8769, 8.4925) knots 0 0 0 1 2 2 2
  line L50 (149.8769, 8.4925) -> (149.8769, 7.8025)
  line L51 (149.8769, 7.8025) -> (149.8282, 7.8025)
  spline S36 degree 2 poles (149.8282, 7.8025) (149.7201, 7.8966) (149.4936, 8.0674) (149.2846, 8.1649) knots 0 0 0 1 2 2 2
  spline S37 degree 2 poles (149.2846, 8.1649) (149.1103, 8.2521) (148.6608, 8.3671) (148.403, 8.3671) knots 0 0 0 1 2 2 2
  spline S38 degree 2 poles (148.403, 8.3671) (147.7827, 8.3671) (147.0161, 7.4332) (147.0161, 6.6561) knots 0 0 0 1 2 2 2
  spline S39 degree 2 poles (147.0161, 6.6561) (147.0161, 6.224) (147.2182, 5.5759) (147.4098, 5.3529) knots 0 0 0 1 2 2 2
  spline S40 degree 2 poles (147.4098, 5.3529) (147.5945, 5.1299) (148.1172, 4.8964) (148.4448, 4.8964) knots 0 0 0 1 2 2 2
  spline S41 degree 2 poles (148.4448, 4.8964) (148.6852, 4.8964) (149.1661, 4.9661) (149.3299, 5.0358) knots 0 0 0 1 2 2 2
  line L52 (149.3299, 5.0358) -> (149.3299, 6.1474)
  line L53 (149.3299, 6.1474) -> (148.3333, 6.1474)
  line L54 (148.3333, 6.1474) -> (148.3333, 6.6491)
  line L55 (148.3333, 6.6491) -> (149.8944, 6.6491)
  line L56 (149.8944, 6.6491) -> (149.8944, 4.7709)
  spline S42 degree 2 poles (149.8944, 4.7709) (149.7863, 4.7222) (149.417, 4.5723) (149.2602, 4.527) knots 0 0 0 1 2 2 2
  spline S43 degree 2 poles (149.2602, 4.527) (149.0476, 4.4643) (148.7061, 4.4016) (148.4657, 4.4016) knots 0 0 0 1 2 2 2
  spline S44 degree 2 poles (152.3684, 4.8267) (152.3022, 4.7779) (152.0792, 4.6037) (151.9747, 4.5514) knots 0 0 0 1 2 2 2
  spline S45 degree 2 poles (151.9747, 4.5514) (151.8318, 4.4748) (151.5635, 4.3946) (151.3196, 4.3946) knots 0 0 0 1 2 2 2
  spline S46 degree 2 poles (151.3196, 4.3946) (151.1209, 4.3946) (150.762, 4.5444) (150.6261, 4.6803) knots 0 0 0 1 2 2 2
  spline S47 degree 2 poles (150.6261, 4.6803) (150.4972, 4.8128) (150.3404, 5.203) (150.3404, 5.4191) knots 0 0 0 1 2 2 2
  spline S48 degree 2 poles (150.3404, 5.4191) (150.3404, 5.7536) (150.6226, 6.2275) (150.9293, 6.3634) knots 0 0 0 1 2 2 2
  spline S49 degree 2 poles (150.9293, 6.3634) (151.2011, 6.4889) (151.9398, 6.5829) (152.3684, 6.6073) knots 0 0 0 1 2 2 2
  line L57 (152.3684, 6.6073) -> (152.3684, 6.7119)
  spline S50 degree 2 poles (152.3684, 6.7119) (152.3684, 6.9) (152.2534, 7.1335) (152.1489, 7.1997) knots 0 0 0 1 2 2 2
  spline S51 degree 2 poles (152.1489, 7.1997) (152.0444, 7.2659) (151.7447, 7.3077) (151.5844, 7.3077) knots 0 0 0 1 2 2 2
  spline S52 degree 2 poles (151.5844, 7.3077) (151.3962, 7.3077) (150.8875, 7.1962) (150.6331, 7.0882) knots 0 0 0 1 2 2 2
  line L58 (150.6331, 7.0882) -> (150.6017, 7.0882)
  line L59 (150.6017, 7.0882) -> (150.6017, 7.6423)
  spline S53 degree 2 poles (150.6017, 7.6423) (150.7516, 7.6841) (151.3126, 7.7886) (151.5879, 7.7886) knots 0 0 0 1 2 2 2
  spline S54 degree 2 poles (151.5879, 7.7886) (151.9224, 7.7886) (152.3789, 7.6841) (152.5601, 7.5482) knots 0 0 0 1 2 2 2
  spline S55 degree 2 poles (152.5601, 7.5482) (152.7378, 7.4158) (152.912, 6.9941) (152.912, 6.691) knots 0 0 0 1 2 2 2
  line L60 (152.912, 6.691) -> (152.912, 4.4852)
  line L61 (152.912, 4.4852) -> (152.3684, 4.4852)
  line L62 (152.3684, 4.4852) -> (152.3684, 4.8267)
  line L63 (152.3684, 5.2797) -> (152.3684, 6.1752)
  spline S56 degree 2 poles (152.3684, 6.1752) (152.1733, 6.1578) (151.5844, 6.0986) (151.3997, 6.0428) knots 0 0 0 1 2 2 2
  spline S57 degree 2 poles (151.3997, 6.0428) (151.1837, 5.9766) (150.9014, 5.7013) (150.9014, 5.4574) knots 0 0 0 1 2 2 2
  spline S58 degree 2 poles (150.9014, 5.4574) (150.9014, 5.1786) (151.215, 4.8964) (151.5147, 4.8964) knots 0 0 0 1 2 2 2
  spline S59 degree 2 poles (151.5147, 4.8964) (151.7691, 4.8964) (152.1872, 5.1159) (152.3684, 5.2797) knots 0 0 0 1 2 2 2
  line L64 (155.3861, 7.13) -> (155.3582, 7.13)
  spline S60 degree 2 poles (155.3582, 7.13) (155.2955, 7.1474) (155.1596, 7.1544) (155.0655, 7.1544) knots 0 0 0 1 2 2 2
  spline S61 degree 2 poles (155.0655, 7.1544) (154.846, 7.1544) (154.4139, 6.9628) (154.2188, 6.7746) knots 0 0 0 1 2 2 2
  line L65 (154.2188, 6.7746) -> (154.2188, 4.4852)
  line L66 (154.2188, 4.4852) -> (153.6752, 4.4852)
  line L67 (153.6752, 4.4852) -> (153.6752, 7.7119)
  line L68 (153.6752, 7.7119) -> (154.2188, 7.7119)
  line L69 (154.2188, 7.7119) -> (154.2188, 7.2311)
  spline S62 degree 2 poles (154.2188, 7.2311) (154.5149, 7.4959) (154.9575, 7.7119) (155.1666, 7.7119) knots 0 0 0 1 2 2 2
  spline S63 degree 2 poles (155.1666, 7.7119) (155.2502, 7.7119) (155.3338, 7.705) (155.3861, 7.6945) knots 0 0 0 1 2 2 2
  line L70 (155.3861, 7.6945) -> (155.3861, 7.13)
  spline S64 degree 2 poles (157.6058, 4.8267) (157.5396, 4.7779) (157.3166, 4.6037) (157.212, 4.5514) knots 0 0 0 1 2 2 2
  spline S65 degree 2 poles (157.212, 4.5514) (157.0692, 4.4748) (156.8008, 4.3946) (156.5569, 4.3946) knots 0 0 0 1 2 2 2
  spline S66 degree 2 poles (156.5569, 4.3946) (156.3583, 4.3946) (155.9994, 4.5444) (155.8635, 4.6803) knots 0 0 0 1 2 2 2
  spline S67 degree 2 poles (155.8635, 4.6803) (155.7346, 4.8128) (155.5778, 5.203) (155.5778, 5.4191) knots 0 0 0 1 2 2 2
  spline S68 degree 2 poles (155.5778, 5.4191) (155.5778, 5.7536) (155.86, 6.2275) (156.1666, 6.3634) knots 0 0 0 1 2 2 2
  spline S69 degree 2 poles (156.1666, 6.3634) (156.4384, 6.4889) (157.1772, 6.5829) (157.6058, 6.6073) knots 0 0 0 1 2 2 2
  line L71 (157.6058, 6.6073) -> (157.6058, 6.7119)
  spline S70 degree 2 poles (157.6058, 6.7119) (157.6058, 6.9) (157.4908, 7.1335) (157.3863, 7.1997) knots 0 0 0 1 2 2 2
  spline S71 degree 2 poles (157.3863, 7.1997) (157.2817, 7.2659) (156.982, 7.3077) (156.8218, 7.3077) knots 0 0 0 1 2 2 2
  spline S72 degree 2 poles (156.8218, 7.3077) (156.6336, 7.3077) (156.1248, 7.1962) (155.8705, 7.0882) knots 0 0 0 1 2 2 2
  line L72 (155.8705, 7.0882) -> (155.8391, 7.0882)
  line L73 (155.8391, 7.0882) -> (155.8391, 7.6423)
  spline S73 degree 2 poles (155.8391, 7.6423) (155.9889, 7.6841) (156.55, 7.7886) (156.8252, 7.7886) knots 0 0 0 1 2 2 2
  spline S74 degree 2 poles (156.8252, 7.7886) (157.1598, 7.7886) (157.6162, 7.6841) (157.7974, 7.5482) knots 0 0 0 1 2 2 2
  spline S75 degree 2 poles (157.7974, 7.5482) (157.9752, 7.4158) (158.1494, 6.9941) (158.1494, 6.691) knots 0 0 0 1 2 2 2
  line L74 (158.1494, 6.691) -> (158.1494, 4.4852)
  line L75 (158.1494, 4.4852) -> (157.6058, 4.4852)
  line L76 (157.6058, 4.4852) -> (157.6058, 4.8267)
  line L77 (157.6058, 5.2797) -> (157.6058, 6.1752)
  spline S76 degree 2 poles (157.6058, 6.1752) (157.4107, 6.1578) (156.8218, 6.0986) (156.6371, 6.0428) knots 0 0 0 1 2 2 2
  spline S77 degree 2 poles (156.6371, 6.0428) (156.421, 5.9766) (156.1388, 5.7013) (156.1388, 5.4574) knots 0 0 0 1 2 2 2
  spline S78 degree 2 poles (156.1388, 5.4574) (156.1388, 5.1786) (156.4524, 4.8964) (156.7521, 4.8964) knots 0 0 0 1 2 2 2
  spline S79 degree 2 poles (156.7521, 4.8964) (157.0064, 4.8964) (157.4246, 5.1159) (157.6058, 5.2797) knots 0 0 0 1 2 2 2
  line L78 (161.4458, 4.4852) -> (160.9022, 4.4852)
  line L79 (160.9022, 4.4852) -> (160.9022, 6.3251)
  spline S80 degree 2 poles (160.9022, 6.3251) (160.9022, 6.5481) (160.8604, 6.9314) (160.7977, 7.0464) knots 0 0 0 1 2 2 2
  spline S81 degree 2 poles (160.7977, 7.0464) (160.7315, 7.1683) (160.4945, 7.2868) (160.2924, 7.2868) knots 0 0 0 1 2 2 2
  spline S82 degree 2 poles (160.2924, 7.2868) (160.0903, 7.2868) (159.6617, 7.0708) (159.4561, 6.8966) knots 0 0 0 1 2 2 2
  line L80 (159.4561, 6.8966) -> (159.4561, 4.4852)
  line L81 (159.4561, 4.4852) -> (158.9125, 4.4852)
  line L82 (158.9125, 4.4852) -> (158.9125, 7.7119)
  line L83 (158.9125, 7.7119) -> (159.4561, 7.7119)
  line L84 (159.4561, 7.7119) -> (159.4561, 7.353)
  spline S83 degree 2 poles (159.4561, 7.353) (159.7, 7.5726) (160.1705, 7.8025) (160.4353, 7.8025) knots 0 0 0 1 2 2 2
  spline S84 degree 2 poles (160.4353, 7.8025) (160.9092, 7.8025) (161.4458, 7.1753) (161.4458, 6.5795) knots 0 0 0 1 2 2 2
  line L85 (161.4458, 6.5795) -> (161.4458, 4.4852)
  spline S85 degree 2 poles (162.3239, 3.9695) (162.3797, 3.9451) (162.5923, 3.8684) (162.7282, 3.8371) knots 0 0 0 1 2 2 2
  spline S86 degree 2 poles (162.7282, 3.8371) (162.878, 3.7987) (163.1324, 3.7534) (163.2822, 3.7534) knots 0 0 0 1 2 2 2
  spline S87 degree 2 poles (163.2822, 3.7534) (163.5331, 3.7534) (163.8816, 3.8859) (163.9791, 4.0043) knots 0 0 0 1 2 2 2
  spline S88 degree 2 poles (163.9791, 4.0043) (164.0732, 4.1228) (164.1464, 4.4329) (164.1464, 4.6316) knots 0 0 0 1 2 2 2
  line L86 (164.1464, 4.6316) -> (164.1464, 4.9138)
  spline S89 degree 2 poles (164.1464, 4.9138) (163.9269, 4.7222) (163.5052, 4.541) (163.1881, 4.541) knots 0 0 0 1 2 2 2
  spline S90 degree 2 poles (163.1881, 4.541) (162.6376, 4.541) (161.9859, 5.3598) (161.9859, 6.1299) knots 0 0 0 1 2 2 2
  spline S91 degree 2 poles (161.9859, 6.1299) (161.9859, 6.5307) (162.2124, 7.1509) (162.4006, 7.3705) knots 0 0 0 1 2 2 2
  spline S92 degree 2 poles (162.4006, 7.3705) (162.5818, 7.576) (163.0801, 7.8025) (163.3449, 7.8025) knots 0 0 0 1 2 2 2
  spline S93 degree 2 poles (163.3449, 7.8025) (163.5958, 7.8025) (163.9617, 7.6841) (164.1464, 7.576) knots 0 0 0 1 2 2 2
  line L87 (164.1464, 7.576) -> (164.1778, 7.7119)
  line L88 (164.1778, 7.7119) -> (164.69, 7.7119)
  line L89 (164.69, 7.7119) -> (164.69, 4.8546)
  spline S94 degree 2 poles (164.69, 4.8546) (164.69, 4.0322) (163.9756, 3.2656) (163.2404, 3.2656) knots 0 0 0 1 2 2 2
  spline S95 degree 2 poles (163.2404, 3.2656) (163.0034, 3.2656) (162.5086, 3.3423) (162.2961, 3.405) knots 0 0 0 1 2 2 2
  line L90 (162.2961, 3.405) -> (162.2961, 3.9695)
  line L91 (162.2961, 3.9695) -> (162.3239, 3.9695)
  line L92 (164.1464, 5.3598) -> (164.1464, 7.1335)
  spline S96 degree 2 poles (164.1464, 7.1335) (163.9443, 7.2311) (163.6028, 7.3147) (163.432, 7.3147) knots 0 0 0 1 2 2 2
  spline S97 degree 2 poles (163.432, 7.3147) (163.0209, 7.3147) (162.547, 6.7084) (162.547, 6.1404) knots 0 0 0 1 2 2 2
  spline S98 degree 2 poles (162.547, 6.1404) (162.547, 5.6038) (162.9059, 5.0427) (163.3101, 5.0427) knots 0 0 0 1 2 2 2
  spline S99 degree 2 poles (163.3101, 5.0427) (163.5226, 5.0427) (163.9687, 5.21) (164.1464, 5.3598) knots 0 0 0 1 2 2 2
  spline S100 degree 2 poles (168.1293, 6.0986) (168.1293, 5.2832) (167.3453, 4.3946) (166.6902, 4.3946) knots 0 0 0 1 2 2 2
  spline S101 degree 2 poles (166.6902, 4.3946) (166.0176, 4.3946) (165.2475, 5.3111) (165.2475, 6.0986) knots 0 0 0 1 2 2 2
  spline S102 degree 2 poles (165.2475, 6.0986) (165.2475, 6.907) (166.042, 7.8025) (166.6902, 7.8025) knots 0 0 0 1 2 2 2
  spline S103 degree 2 poles (166.6902, 7.8025) (167.3453, 7.8025) (168.1293, 6.9105) (168.1293, 6.0986) knots 0 0 0 1 2 2 2
  spline S104 degree 2 poles (167.5683, 6.0986) (167.5683, 6.7258) (167.1118, 7.3356) (166.6902, 7.3356) knots 0 0 0 1 2 2 2
  spline S105 degree 2 poles (166.6902, 7.3356) (166.2685, 7.3356) (165.8085, 6.7258) (165.8085, 6.0986) knots 0 0 0 1 2 2 2
  spline S106 degree 2 poles (165.8085, 6.0986) (165.8085, 5.4888) (166.2685, 4.8615) (166.6902, 4.8615) knots 0 0 0 1 2 2 2
  spline S107 degree 2 poles (166.6902, 4.8615) (167.1083, 4.8615) (167.5683, 5.4783) (167.5683, 6.0986) knots 0 0 0 1 2 2 2
  line L93 (171.1957, 4.4852) -> (170.6521, 4.4852)
  line L94 (170.6521, 4.4852) -> (170.6521, 4.8406)
  spline S108 degree 2 poles (170.6521, 4.8406) (170.4013, 4.6211) (169.9517, 4.3946) (169.673, 4.3946) knots 0 0 0 1 2 2 2